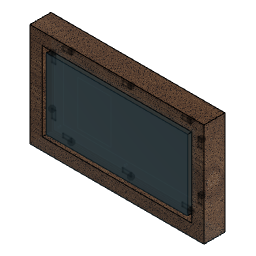
Glowing Square (Autodesk Fusion 360 design; units mm, degrees)
Autodesk Fusion 360 part; units mm, degrees
sketch "Sketch2" plane through (0, 0, 0) normal (0, 1, 0) x (1, 0, 0)
  line L0 (0, 0) -> (256, 0)
  line L1 (256, 0) -> (256, 128)
  line L2 (256, 128) -> (0, 128)
  line L3 (0, 128) -> (0, 0)
  dimension "d1" = 256
  dimension "d2" = 128
  constraint horizontal L0
  constraint vertical L1
  constraint horizontal L2
  constraint vertical L3
  constraint coincident L0.start L3.end
  measures "d1" distance of L0.start L0.end
  measures "d2" distance of L0.start L2.end
extrude "Extrude1" add sketch "Sketch2" along normal blind 14 makes body 1
chamfer "Chamfer1" distance 1 distance2 14 4 edges at (128, 14, 0) (256, 14, -64) (0, 14, -64) (128, 14, -128) measured on face at (85.3333, 14, -85.3333) measured on face at (85.3333, 14, -85.3333) measured on face at (85.3333, 14, -85.3333) measured on face at (85.3333, 14, -85.3333) on bodies 1
sketch "Sketch3" plane through (0, 14, 0) normal (0, 1, 0) x (-1, 0, 0)
  line L0 (-255, -127) -> (-1, -127)
  line L1 (-1, -127) -> (-1, -1)
  line L2 (-1, -1) -> (-255, -1)
  line L3 (-255, -1) -> (-255, -127)
  circle A0 centre (-248, -8) radius 1.5
  circle A1 centre (-128, -8) radius 1.5
  circle A2 centre (-8, -8) radius 1.5
  circle A3 centre (-248, -120) radius 1.5
  circle A4 centre (-128, -120) radius 1.5
  circle A5 centre (-8, -120) radius 1.5
  dimension "d7" = 3
  dimension "d8" = 7
  dimension "d9" = 7
  dimension "d10" = 3
  dimension "d11" = 127
  dimension "d12" = 3
  dimension "d13" = 7
  dimension "d14" = 3
  dimension "d15" = 7
  dimension "d16" = 3
  dimension "d17" = 3
  measures "d7" diameter of A0
  measures "d8" distance of L3 A0.centre
  measures "d9" distance of L2 A0.centre
  measures "d10" diameter of A1
  measures "d11" distance of L3 A1.centre
  measures "d12" diameter of A2
  measures "d13" distance of L1 A2.centre
  measures "d14" diameter of A3
  measures "d15" distance of L0 A3.centre
  measures "d16" diameter of A4
  measures "d17" diameter of A5
extrude "Extrude2" cut sketch "Sketch3" against normal blind 10 contours A0 | A1 | A2 | A3 | A4 | A5 bodies 1
sketch "Sketch4" plane through (0, 14, 0) normal (0, 1, 0) x (-1, 0, 0)
  circle A0 centre (-8, -120) radius 1.5
  circle A1 centre (-248, -8) radius 1.5
  circle A2 centre (-128, -120) radius 1.5
  circle A3 centre (-8, -8) radius 1.5
  circle A4 centre (-128, -8) radius 1.5
  circle A5 centre (-248, -120) radius 1.5
  line L0 (-255, -127) -> (-1, -127)
  line L1 (-1, -127) -> (-1, -1)
  line L2 (-1, -1) -> (-255, -1)
  line L3 (-255, -1) -> (-255, -127)
  line L4 (-103, -24) -> (-43, -24)
  line L5 (-43, -24) -> (-43, -104)
  line L6 (-43, -104) -> (-103, -104)
  line L7 (-103, -104) -> (-103, -24)
  dimension "d20" = 60
  dimension "d21" = 80
  dimension "d22" = 42
  dimension "d23" = 23
  constraint horizontal L4
  constraint vertical L5
  constraint horizontal L6
  constraint vertical L7
  measures "d20" distance of L4.start L4.end
  measures "d21" distance of L4.start L6.end
  measures "d22" distance of L1 L5
  measures "d23" distance of L0 L6
extrude "Extrude3" add sketch "Sketch4" along normal blind 20 contours L4 L5 L6 L7 bodies 1
sketch "Sketch5" plane through (0, 0, 0) normal (0, -1, 0) x (1, 0, 0)
  line L0 (0, 0) -> (0, -128)
  line L1 (0, -128) -> (256, -128)
  line L2 (256, -128) -> (256, 0)
  line L3 (256, 0) -> (0, 0)
copy_body "CutPasteBodies1" bodies 1 removing the originals makes body 2 in component "Display"
sketch "Sketch1" plane through (0, 14, 0) normal (0, 1, 0) x (-1, 0, 0) in component "Display"
  line L0 (-103, -104) -> (-103, -24)
  line L1 (-103, -24) -> (-43, -24)
  line L2 (-43, -24) -> (-43, -104)
  line L3 (-43, -104) -> (-103, -104)
  circle A0 centre (-8, -120) radius 1.5
  circle A1 centre (-248, -8) radius 1.5
  circle A2 centre (-128, -120) radius 1.5
  circle A3 centre (-8, -8) radius 1.5
  circle A4 centre (-128, -8) radius 1.5
  circle A5 centre (-248, -120) radius 1.5
  line L4 (-255, -127) -> (-1, -127)
  line L5 (-1, -127) -> (-1, -1)
  line L6 (-1, -1) -> (-255, -1)
  line L7 (-255, -1) -> (-255, -127)
sketch "Sketch1 (2)" plane through (0, 0, 0) normal (0, 1, 0) x (1, 0, 0) in component "Frame"
  line L0 (-29.5, -29.5) -> (285.5, -29.5)
  line L1 (285.5, -29.5) -> (285.5, 157.5)
  line L2 (285.5, 157.5) -> (-29.5, 157.5)
  line L3 (-29.5, 157.5) -> (-29.5, -29.5)
  line L4 (-7.5, -7.5) -> (263.5, -7.5)
  line L5 (263.5, -7.5) -> (263.5, 135.5)
  line L6 (263.5, 135.5) -> (-7.5, 135.5)
  line L7 (-7.5, 135.5) -> (-7.5, -7.5)
  dimension "d26" = 315
  dimension "d27" = 187
  dimension "d28" = 29.5
  dimension "d29" = 29.5
  dimension "d30" = 22
  dimension "d31" = 22
  dimension "d32" = 22
  dimension "d33" = 22
  constraint horizontal L0
  constraint vertical L1
  constraint horizontal L2
  constraint vertical L3
  constraint horizontal L4
  constraint vertical L5
  constraint horizontal L6
  constraint vertical L7
  measures "d26" distance of L0.start L0.end
  measures "d27" distance of L0.start L2.end
  measures "d28" distance of origin L3
  measures "d29" distance of L0 origin
  measures "d30" distance of L3 L7
  measures "d31" distance of L1 L5
  measures "d32" distance of L0 L4
  measures "d33" distance of L2 L6
extrude "Extrude1'" add sketch "Sketch1 (2)" along normal blind 38 separate body makes body 3 in component "Frame"
sketch "Sketch1 (3)" plane through (0, 14, 0) normal (0, 1, 0) x (-1, 0, 0) in component "Display Mount"
  line L0 (-103, -104) -> (-103, -24)
  line L1 (-103, -24) -> (-43, -24)
  line L2 (-43, -24) -> (-43, -104)
  line L3 (-43, -104) -> (-103, -104)
  circle A0 centre (-8, -120) radius 1.5
  circle A1 centre (-248, -8) radius 1.5
  circle A2 centre (-128, -120) radius 1.5
  circle A3 centre (-8, -8) radius 1.5
  circle A4 centre (-128, -8) radius 1.5
  circle A5 centre (-248, -120) radius 1.5
  line L4 (-255, -127) -> (-1, -127)
  line L5 (-1, -127) -> (-1, -1)
  line L6 (-1, -1) -> (-255, -1)
  line L7 (-255, -1) -> (-255, -127)
  line L8 (-263.5, 7.5) -> (7.5, 7.5)
  line L9 (7.5, 7.5) -> (7.5, -135.5)
  line L10 (7.5, -135.5) -> (-263.5, -135.5)
  line L11 (-263.5, -135.5) -> (-263.5, 7.5)
  line L12 (-256, -128) -> (-256, 0)
  line L13 (-256, 0) -> (0, 0)
  line L14 (-243, -13) -> (-13, -13)
  line L15 (-13, -13) -> (-13, -115)
  line L16 (-13, -115) -> (-243, -115)
  line L17 (-243, -115) -> (-243, -13)
  dimension "d36" = 271
  dimension "d37" = 143
  dimension "d38" = 7.5
  dimension "d39" = 7.5
  dimension "d40" = 5
  dimension "d41" = 5
  dimension "d42" = 5
  dimension "d43" = 5
  dimension "d187" = 256
  dimension "d188" = 128
  constraint horizontal L8
  constraint vertical L9
  constraint horizontal L10
  constraint vertical L11
  constraint horizontal L14
  constraint vertical L15
  constraint horizontal L16
  constraint vertical L17
  measures "d36" distance of L8.start L8.end
  measures "d37" distance of L8.start L10.end
  measures "d38" distance of L11 L12
  measures "d39" distance of L8 L13
  measures "d40" distance of A1.centre L17
  measures "d41" distance of A1.centre L14
  measures "d42" distance of A3.centre L15
  measures "d43" distance of A0.centre L16
  measures "d187" distance of L12.end L13.end
  measures "d188" distance of L12.start L12.end
extrude "Extrude1''" add sketch "Sketch1 (3)" along normal blind 4 separate body contours L4 L5 L6 L7 | L8 L9 L10 L11 makes body 4 in component "Display Mount"
sketch "Sketch2 (2)" plane through (0, 18, 0) normal (0, 1, 0) x (-1, 0, 0) in component "Display Mount"
  circle A0 centre (-8, -8) radius 1.5
  circle A1 centre (-128, -8) radius 1.5
  circle A2 centre (-248, -120) radius 1.5
  circle A3 centre (-8, -120) radius 1.5
  circle A4 centre (-248, -8) radius 1.5
  line L0 (-13, -115) -> (-243, -115)
  line L1 (-243, -115) -> (-243, -13)
  line L2 (-243, -13) -> (-13, -13)
  line L3 (-13, -13) -> (-13, -115)
  circle A5 centre (-128, -120) radius 1.5
  line L4 (-263.5, -135.5) -> (7.5, -135.5)
  line L5 (7.5, -135.5) -> (7.5, 7.5)
  line L6 (7.5, 7.5) -> (-263.5, 7.5)
  line L7 (-263.5, 7.5) -> (-263.5, -135.5)
  line L8 (-243.5, 7.5) -> (-228.5, 7.5)
  line L9 (-228.5, 7.5) -> (-228.5, 1.5)
  line L10 (-228.5, 1.5) -> (-243.5, 1.5)
  line L11 (-243.5, 1.5) -> (-243.5, 7.5)
  line L12 (-27.5, 7.5) -> (-12.5, 7.5)
  line L13 (-12.5, 7.5) -> (-12.5, 1.5)
  line L14 (-12.5, 1.5) -> (-27.5, 1.5)
  line L15 (-27.5, 1.5) -> (-27.5, 7.5)
  line L16 (-263.5, -12.5) -> (-257.5, -12.5)
  line L17 (-257.5, -12.5) -> (-257.5, -27.5)
  line L18 (-257.5, -27.5) -> (-263.5, -27.5)
  line L19 (-263.5, -27.5) -> (-263.5, -12.5)
  line L20 (-243.5, -135.5) -> (-228.5, -135.5)
  line L21 (-228.5, -135.5) -> (-228.5, -129.5)
  line L22 (-228.5, -129.5) -> (-243.5, -129.5)
  line L23 (-243.5, -129.5) -> (-243.5, -135.5)
  line L24 (7.5, -12.5) -> (1.5, -12.5)
  line L25 (1.5, -12.5) -> (1.5, -27.5)
  line L26 (1.5, -27.5) -> (7.5, -27.5)
  line L27 (7.5, -27.5) -> (7.5, -12.5)
  line L28 (-27.5, -135.5) -> (-12.5, -135.5)
  line L29 (-12.5, -135.5) -> (-12.5, -129.5)
  line L30 (-12.5, -129.5) -> (-27.5, -129.5)
  line L31 (-27.5, -129.5) -> (-27.5, -135.5)
  line L32 (-135.5, 7.5) -> (-120.5, 7.5)
  line L33 (-120.5, 7.5) -> (-120.5, 1.5)
  line L34 (-120.5, 1.5) -> (-135.5, 1.5)
  line L35 (-135.5, 1.5) -> (-135.5, 7.5)
  line L36 (-135.5, -135.5) -> (-120.5, -135.5)
  line L37 (-120.5, -135.5) -> (-120.5, -129.5)
  line L38 (-120.5, -129.5) -> (-135.5, -129.5)
  line L39 (-135.5, -129.5) -> (-135.5, -135.5)
  line L40 (-263.5, -100.5) -> (-257.5, -100.5)
  line L41 (-257.5, -100.5) -> (-257.5, -115.5)
  line L42 (-257.5, -115.5) -> (-263.5, -115.5)
  line L43 (-263.5, -115.5) -> (-263.5, -100.5)
  line L44 (7.5, -100.5) -> (1.5, -100.5)
  line L45 (1.5, -100.5) -> (1.5, -115.5)
  line L46 (1.5, -115.5) -> (7.5, -115.5)
  line L47 (7.5, -115.5) -> (7.5, -100.5)
  dimension "d46" = 15
  dimension "d47" = 6
  dimension "d48" = 20
  dimension "d49" = 15
  dimension "d50" = 6
  dimension "d51" = 20
  dimension "d52" = 6
  dimension "d53" = 15
  dimension "d54" = 20
  dimension "d55" = 15
  dimension "d56" = 6
  dimension "d57" = 20
  dimension "d58" = 6
  dimension "d59" = 15
  dimension "d60" = 20
  dimension "d61" = 15
  dimension "d62" = 6
  dimension "d63" = 20
  dimension "d155" = 15
  dimension "d156" = 6
  dimension "d157" = 128
  dimension "d158" = 6
  dimension "d159" = 15
  dimension "d160" = 128
  dimension "d161" = 15
  dimension "d162" = 20
  dimension "d163" = 20
  dimension "d164" = 15
  dimension "d165" = 6
  dimension "d189" = 6
  constraint horizontal L8
  constraint vertical L9
  constraint horizontal L10
  constraint vertical L11
  constraint coincident L6 L8.start
  constraint horizontal L12
  constraint vertical L13
  constraint horizontal L14
  constraint vertical L15
  constraint coincident L6 L12.start
  constraint horizontal L16
  constraint vertical L17
  constraint horizontal L18
  constraint vertical L19
  constraint coincident L7 L16.start
  constraint horizontal L20
  constraint vertical L21
  constraint horizontal L22
  constraint vertical L23
  constraint coincident L4 L20.start
  constraint horizontal L24
  constraint vertical L25
  constraint horizontal L26
  constraint vertical L27
  constraint coincident L5 L24.start
  constraint horizontal L28
  constraint vertical L29
  constraint horizontal L30
  constraint vertical L31
  constraint coincident L4 L28.start
  constraint horizontal L32
  constraint vertical L33
  constraint horizontal L34
  constraint vertical L35
  constraint coincident L6 L32.start
  constraint horizontal L36
  constraint vertical L37
  constraint horizontal L38
  constraint vertical L39
  constraint coincident L4 L36.start
  constraint horizontal L40
  constraint vertical L41
  constraint horizontal L42
  constraint vertical L43
  constraint coincident L7 L40.start
  constraint horizontal L44
  constraint vertical L45
  constraint horizontal L46
  constraint vertical L47
  constraint coincident L5 L44.start
  measures "d46" distance of L8.start L8.end
  measures "d47" distance of L8.start L10.end
  measures "d48" distance of L7 L11
  measures "d49" distance of L12.start L12.end
  measures "d50" distance of L12.start L14.end
  measures "d51" distance of L5 L13
  measures "d52" distance of L16.start L16.end
  measures "d53" distance of L16.start L18.end
  measures "d54" distance of L6 L16
  measures "d55" distance of L20.start L20.end
  measures "d56" distance of L20.start L22.end
  measures "d57" distance of L7 L23
  measures "d58" distance of L24.start L24.end
  measures "d59" distance of L24.start L26.end
  measures "d60" distance of L6 L24
  measures "d61" distance of L28.start L28.end
  measures "d62" distance of L28.start L30.end
  measures "d63" distance of L5 L29
  measures "d155" distance of L32.start L32.end
  measures "d156" distance of L32.start L34.end
  measures "d157" distance of L7 L35
  measures "d158" distance of L36.start L38.end
  measures "d159" distance of L37.end L38.end
  measures "d160" distance of L7 L36.start
  measures "d161" distance of L40.start L42.end
  measures "d162" distance of L4 L42.end
  measures "d163" distance of L4 L46
  measures "d164" distance of L44.start L46.end
  measures "d165" distance of L44.start L44.end
  measures "d189" distance of L40.start L40.end
extrude "Extrude2'" add sketch "Sketch2 (2)" along normal blind 15 contours L4 L20 L21 L22 L23 | L7 L40 L41 L42 L43 | L4 L36 L37 L38 L39 | L7 L16 L17 L18 L19 | L4 L28 L29 L30 L31 | L6 L8 L9 L10 L11 | L5 L44 L45 L46 L47 | L6 L32 L33 L34 L35 | L5 L24 L25 L26 L27 | L6 L12 L13 L14 L15 bodies 4 in component "Display Mount"
fillet "Fillet1" radius 2 30 edges at (228.5, 18, 4.5) (12.5, 18, 4.5) (243.5, 18, 4.5) (27.5, 18, 4.5) (-4.5, 18, -27.5) (-4.5, 18, -12.5) (236, 18, 1.5) (20, 18, 1.5) (257.5, 18, -20) (260.5, 18, -27.5) (-1.5, 18, -20) (20, 18, -129.5) (27.5, 18, -132.5) (236, 18, -129.5) (228.5, 18, -132.5) (260.5, 18, -12.5) (12.5, 18, -132.5) (243.5, 18, -132.5) (128, 18, 1.5) (260.5, 18, -115.5) (-4.5, 18, -115.5) (120.5, 18, 4.5) (257.5, 18, -108) (120.5, 18, -132.5) (128, 18, -129.5) (-4.5, 18, -100.5) (260.5, 18, -100.5) (135.5, 18, 4.5) (-1.5, 18, -108) (135.5, 18, -132.5) on bodies 4 in component "Display Mount"
hole "Hole1" at (20, 26.5, 1.5) direction (0, 0, 1) diameter 4 depth 6 tip angle 180 countersink diameter 6.6 countersink angle 90 bodies 4 in component "Display Mount"
hole "Hole2" at (236, 26.5, 1.5) direction (0, 0, 1) diameter 4 depth 6 tip angle 180 countersink diameter 6.6 countersink angle 90 bodies 4 in component "Display Mount"
hole "Hole3" at (257.5, 26.5, -20) direction (1, 0, 0) diameter 4 depth 6 tip angle 180 countersink diameter 6.6 countersink angle 90 bodies 4 in component "Display Mount"
hole "Hole4" at (236, 26.5, -129.5) direction (0, 0, -1) diameter 4 depth 6 tip angle 180 countersink diameter 6.6 countersink angle 90 bodies 4 in component "Display Mount"
hole "Hole5" at (20, 26.5, -129.5) direction (0, 0, -1) diameter 4 depth 6 tip angle 180 countersink diameter 6.6 countersink angle 90 bodies 4 in component "Display Mount"
hole "Hole6" at (-1.5, 26.5, -20) direction (-1, 0, 0) diameter 4 depth 6 tip angle 180 countersink diameter 6.6 countersink angle 90 bodies 4 in component "Display Mount"
sketch "Sketch1 (4)" plane through (0, 38, 0) normal (0, 1, 0) x (-1, 0, 0) in component "Wall Mount"
  line L0 (7.5, 7.5) -> (7.5, -135.5)
  line L1 (7.5, -135.5) -> (-263.5, -135.5)
  line L2 (-263.5, -135.5) -> (-263.5, 7.5)
  line L3 (-263.5, 7.5) -> (7.5, 7.5)
  line L4 (29.5, -157.5) -> (29.5, 29.5)
  line L5 (29.5, 29.5) -> (-285.5, 29.5)
  line L6 (-285.5, 29.5) -> (-285.5, -157.5)
  line L7 (-285.5, -157.5) -> (29.5, -157.5)
  line L8 (-273.5, 17.5) -> (17.5, 17.5)
  line L9 (17.5, 17.5) -> (17.5, -145.5)
  line L10 (17.5, -145.5) -> (-273.5, -145.5)
  line L11 (-273.5, -145.5) -> (-273.5, 17.5)
  dimension "d97" = 291
  dimension "d98" = 163
  dimension "d99" = 10
  dimension "d100" = 10
  constraint horizontal L8
  constraint vertical L9
  constraint horizontal L10
  constraint vertical L11
  measures "d97" distance of L8.start L8.end
  measures "d98" distance of L8.start L10.end
  measures "d99" distance of L3 L8
  measures "d100" distance of L2 L11
extrude "Extrude1'''" add sketch "Sketch1 (4)" along normal blind 2 separate body contours L0 L1 L2 L3 | L8 L9 L10 L11 makes body 5 in component "Wall Mount"
sketch "Sketch2 (3)" plane through (0, 0, -157.5) normal (0, 0, -1) x (1, 0, 0) in component "Frame"
  line L0 (285.5, 0) -> (-29.5, 0)
  line L1 (-29.5, 0) -> (-29.5, -38)
  line L2 (-29.5, -38) -> (285.5, -38)
  line L3 (285.5, -38) -> (285.5, 0)
sketch "Sketch3 (2)" plane through (0, 0, -157.5) normal (0, 0, -1) x (1, 0, 0) in component "Frame"
  circle A0 centre (128, -34) radius 4
  line L0 (-29.5, 0) -> (-29.5, -38)
  line L1 (-29.5, -38) -> (285.5, -38)
  line L2 (132, -38) -> (124, -38)
  line L3 (124, -38) -> (124, -34)
  line L4 (124, -34) -> (132, -34)
  line L5 (132, -34) -> (132, -38)
  line L6 (285.5, 0) -> (-29.5, 0)
  dimension "d106" = 8
  dimension "d107" = 157.5
  dimension "d108" = 4
  dimension "d109" = 8
  dimension "d190" = 315
  constraint horizontal L2
  constraint vertical L3
  constraint horizontal L4
  constraint vertical L5
  constraint coincident A0 L3.end
  constraint coincident L1 L2.start
  measures "d106" diameter of A0
  measures "d107" distance of A0.centre L0
  measures "d108" distance of A0.centre L1
  measures "d109" distance of L3.end L4.end
  measures "d190" distance of L6.start L0.start
extrude "Extrude2''" cut sketch "Sketch3 (2)" against normal blind 22 bodies 3 in component "Frame"
sketch "Sketch3 (3)" plane through (0, 38, 0) normal (0, -1, 0) x (1, 0, 0) in component "Wall Mount"
  line L0 (-17.5, -145.5) -> (273.5, -145.5)
  line L1 (273.5, -145.5) -> (273.5, 17.5)
  line L2 (273.5, 17.5) -> (-17.5, 17.5)
  line L3 (-17.5, 17.5) -> (-17.5, -145.5)
  line L4 (-7.5, 7.5) -> (258.5, 7.5)
  line L5 (258.5, 7.5) -> (258.5, -130.5)
  line L6 (258.5, -130.5) -> (-7.5, -130.5)
  line L7 (-7.5, -130.5) -> (-7.5, 7.5)
  dimension "d140" = 266
  dimension "d141" = 138
  dimension "d142" = 10
  dimension "d143" = 10
  constraint horizontal L4
  constraint vertical L5
  constraint horizontal L6
  constraint vertical L7
  measures "d140" distance of L4.start L4.end
  measures "d141" distance of L4.start L6.end
  measures "d142" distance of L2 L4
  measures "d143" distance of L3 L7
extrude "Extrude3'" add sketch "Sketch3 (3)" along normal blind 2 contours L4 L5 L6 L7 bodies 5 in component "Wall Mount"
sketch "Sketch2 (4)" plane through (0, 40, 0) normal (0, 1, 0) x (-1, 0, 0) in component "Wall Mount"
  line L0 (-273.5, -145.5) -> (17.5, -145.5)
  line L1 (17.5, -145.5) -> (17.5, 17.5)
  line L2 (17.5, 17.5) -> (-273.5, 17.5)
  line L3 (-273.5, 17.5) -> (-273.5, -145.5)
  circle A0 centre (-268.5, 12.5) radius 2
  circle A1 centre (12.5, 12.5) radius 2
  circle A2 centre (-268.5, -140.5) radius 2
  circle A3 centre (12.5, -140.5) radius 2
  circle A4 centre (-128, -22.5) radius 7
  circle A5 centre (-128, -15.5) radius 3.5
  dimension "d112" = 4
  dimension "d113" = 5
  dimension "d114" = 5
  dimension "d115" = 4
  dimension "d116" = 5
  dimension "d117" = 5
  dimension "d118" = 4
  dimension "d119" = 5
  dimension "d120" = 5
  dimension "d121" = 4
  dimension "d122" = 5
  dimension "d123" = 5
  dimension "d134" = 14
  dimension "d135" = 145.5
  dimension "d136" = 40
  dimension "d146" = 7
  constraint coincident A4 A5.centre
  measures "d112" diameter of A0
  measures "d113" distance of L2 A0.centre
  measures "d114" distance of L3 A0.centre
  measures "d115" diameter of A1
  measures "d116" distance of L1 A1.centre
  measures "d117" distance of L2 A1.centre
  measures "d118" diameter of A2
  measures "d119" distance of L0 A2.centre
  measures "d120" distance of L3 A2.centre
  measures "d121" diameter of A3
  measures "d122" distance of L1 A3.centre
  measures "d123" distance of L0 A3.centre
  measures "d134" diameter of A4
  measures "d135" distance of L3 A4.centre
  measures "d136" distance of L2 A4.centre
  measures "d146" diameter of A5
extrude "Extrude2'''" cut sketch "Sketch2 (4)" against normal blind 10 contours A4 A5 | A4 A5 | A4 A5 bodies 5 in component "Wall Mount"
hole "Hole2'" [suppressed] in component "Frame"
hole "Hole1'" at (268.5, 40, 12.5) at (-12.5, 40, 12.5) at (-12.5, 40, -140.5) at (268.5, 40, -140.5) direction (0, -1, 0) diameter 4 depth 2 tip angle 180 countersink diameter 6.6 countersink angle 90 bodies 5 in component "Wall Mount"
hole "Hole7" at (128, 26.5, 1.5) direction (0, 0, 1) diameter 4 depth 6 tip angle 118 countersink diameter 6.6 countersink angle 90 bodies 4 in component "Display Mount"
hole "Hole8" at (128, 26.5, -129.5) direction (0, 0, -1) diameter 4 depth 6 tip angle 180 countersink diameter 6.6 countersink angle 90 bodies 4 in component "Display Mount"
hole "Hole9" at (257.5, 26.5, -108) direction (1, 0, 0) diameter 4 depth 6 tip angle 180 countersink diameter 6.6 countersink angle 90 bodies 4 in component "Display Mount"
hole "Hole10" at (-1.5, 26.5, -108) direction (-1, 0, 0) diameter 4 depth 6 tip angle 180 countersink diameter 6.6 countersink angle 90 bodies 4 in component "Display Mount"
sketch "Sketch3 (4)" plane through (0, 18, 0) normal (0, 1, 0) x (-1, 0, 0) in component "Display Mount"
  line L0 (-245.5, -135.5) -> (-245.5, -127.5)
  line L1 (-245.5, -127.5) -> (-226.5, -127.5)
  line L2 (-226.5, -127.5) -> (-226.5, -135.5)
  line L3 (-118.5, -135.5) -> (-29.5, -135.5)
  line L4 (-29.5, -135.5) -> (-29.5, -127.5)
  line L5 (-29.5, -127.5) -> (-10.5, -127.5)
  line L6 (-10.5, -127.5) -> (-10.5, -135.5)
  line L7 (-10.5, -135.5) -> (7.5, -135.5)
  line L8 (7.5, -135.5) -> (7.5, -117.5)
  line L9 (7.5, -29.5) -> (-0.5, -29.5)
  line L10 (-0.5, -29.5) -> (-0.5, -10.5)
  line L11 (-0.5, -10.5) -> (7.5, -10.5)
  line L12 (7.5, -10.5) -> (7.5, 7.5)
  line L13 (7.5, 7.5) -> (-10.5, 7.5)
  line L14 (-10.5, 7.5) -> (-10.5, -0.5)
  line L15 (-10.5, -0.5) -> (-29.5, -0.5)
  line L16 (-29.5, -0.5) -> (-29.5, 7.5)
  line L17 (-29.5, 7.5) -> (-118.5, 7.5)
  line L18 (-226.5, 7.5) -> (-226.5, -0.5)
  line L19 (-226.5, -0.5) -> (-245.5, -0.5)
  line L20 (-245.5, -0.5) -> (-245.5, 7.5)
  line L21 (-245.5, 7.5) -> (-263.5, 7.5)
  line L22 (-263.5, 7.5) -> (-263.5, -10.5)
  line L23 (-263.5, -10.5) -> (-255.5, -10.5)
  line L24 (-255.5, -10.5) -> (-255.5, -29.5)
  line L25 (-255.5, -29.5) -> (-263.5, -29.5)
  line L26 (-263.5, -29.5) -> (-263.5, -98.5)
  line L27 (-263.5, -135.5) -> (-245.5, -135.5)
  circle A0 centre (-128, -120) radius 1.5
  line L28 (-13, -115) -> (-243, -115)
  line L29 (-243, -115) -> (-243, -13)
  line L30 (-243, -13) -> (-13, -13)
  line L31 (-13, -13) -> (-13, -115)
  circle A1 centre (-248, -8) radius 1.5
  circle A2 centre (-8, -120) radius 1.5
  circle A3 centre (-248, -120) radius 1.5
  circle A4 centre (-128, -8) radius 1.5
  circle A5 centre (-8, -8) radius 1.5
  circle A6 centre (-26, -9.5) radius 2.25
  line L32 (-23.75, -9.5) -> (-23.75, -13)
  line L33 (-28.25, -9.5) -> (-28.25, -13)
  circle A7 centre (-230, -118.5) radius 2.25
  line L34 (-227.75, -118.5) -> (-227.75, -115)
  line L35 (-232.25, -118.5) -> (-232.25, -115)
  line L36 (-118.5, -127.5) -> (-118.5, -135.5)
  line L37 (7.5, -117.5) -> (-0.5, -117.5)
  line L38 (-0.5, -117.5) -> (-0.5, -98.5)
  line L39 (-0.5, -98.5) -> (7.5, -98.5)
  line L40 (7.5, -98.5) -> (7.5, -29.5)
  line L41 (-118.5, 7.5) -> (-118.5, -0.5)
  line L42 (-118.5, -0.5) -> (-137.5, -0.5)
  line L43 (-137.5, -0.5) -> (-137.5, 7.5)
  line L44 (-137.5, 7.5) -> (-226.5, 7.5)
  line L45 (-263.5, -98.5) -> (-255.5, -98.5)
  line L46 (-255.5, -98.5) -> (-255.5, -117.5)
  line L47 (-255.5, -117.5) -> (-263.5, -117.5)
  line L48 (-263.5, -117.5) -> (-263.5, -135.5)
  line L49 (-226.5, -135.5) -> (-137.5, -135.5)
  line L50 (-137.5, -135.5) -> (-137.5, -127.5)
  line L51 (-137.5, -127.5) -> (-118.5, -127.5)
  dimension "d147" = 13
  dimension "d148" = 3.5
  dimension "d151" = 4.5
  dimension "d152" = 4.5
  dimension "d153" = 13
  dimension "d154" = 3.5
  constraint coincident A6 L32.start
  constraint coincident L30 L32.end
  constraint tangent A6 L32
  constraint perpendicular L30 L32
  constraint coincident A6 L33.start
  constraint coincident L30 L33.end
  constraint tangent A6 L33
  constraint perpendicular L30 L33
  constraint coincident A7 L34.start
  constraint coincident L28 L34.end
  constraint tangent A7 L34
  constraint perpendicular L28 L34
  constraint coincident A7 L35.start
  constraint coincident L28 L35.end
  constraint tangent A7 L35
  constraint perpendicular L28 L35
  measures "d147" distance of L31 A6.centre
  measures "d148" distance of L30 A6.centre
  measures "d151" diameter of A6
  measures "d152" diameter of A7
  measures "d153" distance of L29 A7.centre
  measures "d154" distance of L28 A7.centre
extrude "Extrude3''" cut sketch "Sketch3 (4)" against normal blind 10 contours L28 A7 L34 L35 | A7 | L30 A6 L32 L33 | A6 bodies 4 in component "Display Mount"
chamfer "Chamfer1'" distance 4 angle 45 20 edges at (135.5, 33, 4.5) (120.5, 33, 4.5) (27.5, 33, 4.5) (12.5, 33, 4.5) (-4.5, 33, -12.5) (-4.5, 33, -27.5) (120.5, 33, -132.5) (135.5, 33, -132.5) (-4.5, 33, -100.5) (-4.5, 33, -115.5) (12.5, 33, -132.5) (27.5, 33, -132.5) (228.5, 33, -132.5) (243.5, 33, -132.5) (260.5, 33, -115.5) (260.5, 33, -100.5) (260.5, 33, -27.5) (260.5, 33, -12.5) (243.5, 33, 4.5) (228.5, 33, 4.5) on bodies 4 in component "Display Mount"
component "Display" placed x (1, 0, 0) y (0, 1, 0) z (0, 0, 1) at (0, 0, 0)
component "Frame" placed x (1, 0, 0) y (0, 1, 0) z (0, 0, 1) at (0, 0, 0)
component "Display Mount" placed x (1, 0, 0) y (0, 1, 0) z (0, 0, 1) at (0, 0, 0) in component "Display"
component "Wall Mount" placed x (1, 0, 0) y (0, 1, 0) z (0, 0, 1) at (0, 0, 0) in component "Frame"
equation "d26 = 310 mm + 5 mm"
equation "d27 = 182 mm + 5 mm"
equation "d28 = 32 mm - 2.5 mm"
equation "d29 = 32 mm - 2.5 mm"
equation "d36 = 256.00 mm + d38 * 2"
equation "d37 = 128.00 mm + 2 * ( d39 )"
equation "d39 = d38"
equation "d49 = d46"
equation "d51 = d48"
equation "d53 = d46"
equation "d54 = d48"
equation "d55 = d46"
equation "d57 = d48"
equation "d59 = d46"
equation "d60 = d54"
equation "d61 = d46"
equation "d63 = d51"
equation "d97 = 256 mm + 35 mm"
equation "d98 = 128 mm + 35 mm"
equation "d107 = ( 315 / 2 ) * 1 mm"
equation "d113 = d114"
equation "d116 = d114"
equation "d117 = d114"
equation "d119 = d114"
equation "d120 = d114"
equation "d122 = d114"
equation "d123 = d114"
equation "d135 = ( 291 / 2 ) * 1 mm"
equation "d140 = 286 mm - 20 mm"
equation "d152 = d151"
equation "d153 = d147"
equation "d154 = d148"
equation "d155 = d46"
equation "d156 = d47"
equation "d157 = ( 271 mm - d46 ) / 2"
equation "d158 = d47"
equation "d159 = d46"
equation "d160 = d157"
equation "d161 = d46"
equation "d162 = d54"
equation "d163 = d54"
equation "d164 = d46"
equation "d165 = d47"
equation "d189 = d47"
